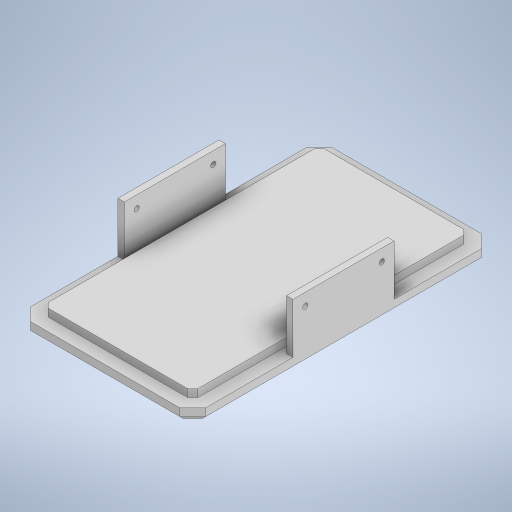
# Autodesk Inventor part: 컨버터 커버
Saved by Autodesk Inventor 2023 (Build 270158000, 158)
## iProperties
Created: 2022-08-19
Part Number: 컨버터 커버
Material: 일반
Document SubType Name: Modeling
Designer: user
Density: 1 g/cm^3
Appearance: 기본값
Author: user
Autodesk Inventor part; units mm, degrees
ref_plane "YZ Plane" through (0, 0, 0) normal (1, 0, 0) x (0, 1, 0)
ref_plane "XZ Plane" through (0, 0, 0) normal (0, 1, 0) x (-1, 0, 0)
ref_plane "XY Plane" through (0, 0, 0) normal (0, 0, 1) x (1, 0, 0)
sketch "스케치1" plane through (0, 0, 0) normal (0, 1, 0) x (-1, 0, 0)
  line L0 (-29.3, -54.1) -> (29.3, -54.1)
  line L1 (29.3, -54.1) -> (29.3, 54.1)
  line L2 (29.3, 54.1) -> (-29.3, 54.1)
  line L3 (-29.3, 54.1) -> (-29.3, -54.1)
  line L4 (-29.3, -54.1) -> (29.3, 54.1) construction
  line L5 (29.3, -54.1) -> (-29.3, 54.1) construction
  line L6 (34.3, 59.1) -> (34.3, -59.1)
  line L7 (34.3, -59.1) -> (-34.3, -59.1)
  line L8 (-34.3, -59.1) -> (-34.3, 59.1)
  line L9 (-34.3, 59.1) -> (34.3, 59.1)
  line L10 (34.3, 19.8) -> (29.3, 19.8)
  line L11 (29.3, 19.8) -> (29.3, -19.8)
  line L12 (29.3, -19.8) -> (34.3, -19.8)
  line L13 (34.3, -19.8) -> (34.3, 19.8)
  line L14 (34.3, 19.8) -> (29.3, -19.8) construction
  line L15 (29.3, 19.8) -> (34.3, -19.8) construction
  line L16 (0, 0) -> (0, -10.2235)
  line L17 (31.8, 19.8) -> (31.8, -19.8)
  line L18 (-34.3, 19.8) -> (-29.3, 19.8)
  line L19 (-29.3, 19.8) -> (-29.3, -19.8)
  line L20 (-29.3, -19.8) -> (-34.3, -19.8)
  line L21 (-34.3, -19.8) -> (-34.3, 19.8)
  line L22 (-34.3, 19.8) -> (-29.3, -19.8) construction
  line L23 (-29.3, 19.8) -> (-34.3, -19.8) construction
  line L24 (-31.8, 19.8) -> (-31.8, -19.8)
  point P0 (31.8, 0)
  point P1 (-31.8, 0)
  point P2 (-34.3, 19.8)
  point P3 (-34.3, -19.8)
  point P4 (34.3, 19.8)
  dimension "d0" = 58.6
  dimension "d1" = 108.2
  dimension "d4" = 5
  dimension "d7" = 39.6
  constraints: 50 end point, 7 symmetric about line, 6 midpoint, 6 parallel, 3 perpendicular, 2 horizontal, 2 point on line, 1 horizontal alignment, 1 vertical, 3 other
  measures "d0" distance of L2.end L1.end
  measures "d1" distance of L1.end L0.end
  measures "d4" distance between parallel lines of L1 L6
  measures "d7" distance between parallel lines of L12 L10
extrude "돌출1" add sketch "스케치1" against normal blind 5
extrude "돌출2" add sketch "스케치1" along normal blind 19.7 contours L20 L8 L18 L24 | L17 L10 L6 L12
chamfer "모따기1" distance 5 angle 45 4 edges at (-34.3, -2.5, 59.1) (34.3, -2.5, 59.1) (34.3, -2.5, -59.1) (-34.3, -2.5, -59.1)
sketch "스케치2" plane through (34.3, 0, -19.8) normal (1, 0, 0) x (0, 0, -1)
  circle A0 centre (-4.8, 15) radius 1
  line L0 (-19.8, 0) -> (-19.8, 7.8444)
  line L1 (-39.6, 19.7) -> (0, 19.7) projected
  line L2 (-39.6, 0) -> (0, 0) projected
  circle A1 centre (-34.8, 15) radius 1
  dimension "d14" = 15
  dimension "d15" = 2
  dimension "d16" = 15
  constraints: 2 centre point, 2 end point, 1 symmetric about line, 1 vertical, 1 other
  measures "d14" distance from line of L0 A0.centre
  measures "d15" diameter of A0
  measures "d16" distance from line of L2 A0.centre
extrude "돌출3" cut sketch "스케치2" against normal up to surface (68.6 mm away)
extrude "돌출4" add sketch "스케치1" along normal blind 3 contours L3 L2 L1 L0
chamfer "모따기2" distance 2 angle 45 4 edges at (-29.3, 1.5, -54.1) (-29.3, 1.5, 54.1) (29.3, 1.5, -54.1) (29.3, 1.5, 54.1)
chamfer "모따기3" distance 2 angle 45 8 edges at (34.3, -5, 0) (31.8, -5, -56.6) (0, -5, -59.1) (-34.3, -5, 0) (-31.8, -5, -56.6) (31.8, -5, 56.6) (0, -5, 59.1) (-31.8, -5, 56.6)
